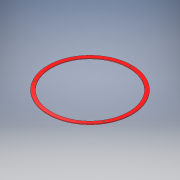
# Autodesk Inventor part: Bearing Spacer
Saved by Autodesk Inventor 2019.4 (Build 234330000, 330)
## iProperties
Created: 2020-01-23
Part Number: Bearing Spacer
Material: Plywood, Finish
Document SubType Name: Modeling
Designer: admin
Density: 0.552 g/cm^3
Appearance: Plywood - New
Mass: 23.2512 g
Surface Area: 348.198 cm^2
Volume: 42.1217 cm^3
Author: admin
Autodesk Inventor part; units mm, degrees
ref_plane "YZ Plane" through (0, 0, 0) normal (1, 0, 0) x (0, 1, 0)
ref_plane "XZ Plane" through (0, 0, 0) normal (0, 1, 0) x (-1, 0, 0)
ref_plane "XY Plane" through (0, 0, 0) normal (0, 0, 1) x (1, 0, 0)
sketch "Sketch1" plane through (0, 0, 0) normal (0, 1, 0) x (-1, 0, 0)
  circle A0 centre (0, 0) radius 160.5
  circle A1 centre (0, 0) radius 147.5
  line L0 (0, -154.7299) -> (-134, 77.3649) construction
  line L1 (-134, 77.3649) -> (134, 77.3649) construction
  line L2 (134, 77.3649) -> (0, -154.7299) construction
  circle A2 centre (0, -154.7299) radius 3
  circle A3 centre (-134, 77.3649) radius 3
  circle A4 centre (134, 77.3649) radius 3
  dimension "d1" = 13
  dimension "d11" = 295
  dimension "d12" = 268
  dimension "d13" = 6
  dimension "d14" = 6
  dimension "d15" = 6
  constraints: 7 coincident, 6 end point, 5 centre point, 1 horizontal, 7 other
  measures "d1" radial gap between concentric circles of A0 A1
  measures "d11" diameter of A1
  measures "d12" distance of L0.end L1.end
  measures "d13" diameter of A2
  measures "d14" diameter of A3
  measures "d15" diameter of A4
extrude "Extrusion1" add sketch "Sketch1" along normal blind 3
body "Solid1"
